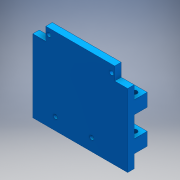
# Autodesk Inventor part: arduinoPlate
Saved by Autodesk Inventor 2016 (Build 200138000, 138)
## iProperties
Created: 2016-06-12
Part Number: arduinoPlate
Material: ABS Plastic
Document SubType Name: Modeling
Designer: hesaon
Density: 1.06 g/cm^3
Appearance: Smooth - White
Author: hesaon
Autodesk Inventor part; units mm, degrees
ref_plane "YZ Plane" through (0, 0, 0) normal (1, 0, 0) x (0, 1, 0)
ref_plane "XZ Plane" through (0, 0, 0) normal (0, 1, 0) x (-1, 0, 0)
ref_plane "XY Plane" through (0, 0, 0) normal (0, 0, 1) x (1, 0, 0)
sketch "Sketch1" plane through (0, 0, 0) normal (0, 1, 0) x (-1, 0, 0)
  line L0 (0, 0) -> (73, 0)
  line L1 (73, 0) -> (73, -56)
  line L2 (73, -56) -> (0, -56)
  line L3 (0, -56) -> (0, 0)
  dimension "d0" = 73
  dimension "d1" = 56
  constraints: 8 end point, 2 parallel, 1 horizontal, 1 perpendicular
  measures "d0" distance of L1.end L2.end
  measures "d1" distance of L0.end L1.end
extrude "Extrusion1" add sketch "Sketch1" along normal blind 5
sketch "Sketch2" plane through (0, 5, 0) normal (0, 1, 0) x (1, 0, 0)
  line L0 (-73, 46) -> (-63, 46)
  line L1 (-63, 46) -> (-63, 36)
  line L2 (-63, 36) -> (-73, 36)
  line L3 (-73, 36) -> (-73, 46)
  line L4 (-10, 46) -> (0, 46)
  line L5 (0, 46) -> (0, 36)
  line L6 (0, 36) -> (-10, 36)
  line L7 (-10, 36) -> (-10, 46)
  line L8 (-73, 20) -> (-63, 20)
  line L9 (-63, 20) -> (-63, 10)
  line L10 (-63, 10) -> (-73, 10)
  line L11 (-73, 10) -> (-73, 20)
  line L12 (-10, 20) -> (0, 20)
  line L13 (0, 20) -> (0, 10)
  line L14 (0, 10) -> (-10, 10)
  line L15 (-10, 10) -> (-10, 20)
  line L16 (-73, 56) -> (-73, 0) projected
  line L17 (0, 0) -> (0, 56) projected
  line L18 (0, 56) -> (-73, 56) projected
  line L19 (-73, 0) -> (0, 0) projected
  dimension "d4" = 10
  dimension "d5" = 10
  dimension "d6" = 10
  dimension "d7" = 10
  dimension "d8" = 10
  dimension "d9" = 10
  dimension "d10" = 10
  dimension "d11" = 10
  dimension "d12" = 10
  dimension "d13" = 10
  dimension "d14" = 10
  dimension "d15" = 10
  constraints: 32 end point, 8 parallel, 4 collinear, 4 horizontal, 4 perpendicular
  measures "d4" distance of L1.end L2.end
  measures "d5" distance of L0.end L1.end
  measures "d6" distance of L5.end L6.end
  measures "d7" distance of L4.end L5.end
  measures "d8" distance of L9.end L10.end
  measures "d9" distance of L8.end L9.end
  measures "d10" distance of L13.end L14.end
  measures "d11" distance of L12.end L13.end
  measures "d12" distance between parallel lines of L18 L0
  measures "d13" distance between parallel lines of L19 L10
  measures "d14" distance between parallel lines of L19 L14
  measures "d15" distance between parallel lines of L18 L4
extrude "Extrusion2" add sketch "Sketch2" along normal blind 10 contours L0 L1 L2 L3 | L8 L9 L10 L11 | L5 L6 L7 L4 | L13 L14 L15 L12
hole "Hole1" at (-68, 10, -46) direction (0, 0, 1) diameter 4.3 end through all
hole "Hole2" at (-5, 10, -46) direction (0, 0, 1) diameter 4.3 end through all
sketch "Sketch4" plane through (0, 0, 0) normal (0, -1, 0) x (1, 0, 0)
  line L0 (-63.15, 19.6) -> (-9.85, 19.6)
  line L1 (-9.85, 19.6) -> (-9.85, -49)
  line L2 (-9.85, -49) -> (-63.15, -49)
  line L3 (-63.15, -49) -> (-63.15, 19.6)
  line L4 (0, -56) -> (-73, -56) projected
  line L5 (-73, 0) -> (-73, -56) projected
  circle A0 centre (-55.55, -46.5) radius 1.6
  circle A1 centre (-27.65, -46.5) radius 1.6
  circle A2 centre (-12.45, 4.3) radius 1.6
  circle A3 centre (-60.65, 5.6) radius 1.6
  point P0 (0, 0)
  dimension "d40" = 53.3
  dimension "d41" = 68.6
  dimension "d42" = 7
  dimension "d43" = 9.85
  dimension "d44" = 3.2
  dimension "d45" = 3.2
  dimension "d46" = 3.2
  dimension "d47" = 3.2
  dimension "d48" = 14
  dimension "d49" = 15.3
  dimension "d50" = 2.5
  dimension "d51" = 7.6
  dimension "d52" = 66.1
  dimension "d53" = 66.1
  dimension "d54" = 27.9
  dimension "d55" = 15.2
  constraints: 8 end point, 4 centre point, 2 parallel, 1 horizontal, 1 perpendicular
  measures "d40" distance of L1.end L2.end
  measures "d41" distance of L0.end L1.end
  measures "d42" distance between parallel lines of L4 L2
  measures "d43" distance between parallel lines of L5 L3
  measures "d44" diameter of A0
  measures "d45" diameter of A1
  measures "d46" diameter of A2
  measures "d47" diameter of A3
  measures "d48" distance from line of L0 A3.centre
  measures "d49" distance from line of L0 A2.centre
  measures "d50" distance from line of L3 A3.centre
  measures "d51" distance from line of L3 A0.centre
  measures "d52" distance from line of L0 A0.centre
  measures "d53" distance from line of L0 A1.centre
  measures "d54" distance of A0.centre A1.centre
  measures "d55" horizontal distance of A1.centre A2.centre
sketch "Sketch5" plane through (-73, 0, 0) normal (0, 0, 1) x (1, 0, 0)
  line L0 (10, 5) -> (63, 5)
  line L1 (63, 5) -> (63, 0)
  line L2 (63, 0) -> (10, 0)
  line L3 (10, 0) -> (10, 5)
  line L4 (73, 0) -> (0, 0) projected
  line L5 (0, 5) -> (73, 5) projected
  line L6 (73, 0) -> (73, 5) projected
  dimension "d56" = 10
  dimension "d57" = 10
  constraints: 8 end point, 2 collinear, 2 parallel, 1 horizontal, 1 perpendicular
  measures "d56" distance of L5.start L0.start
  measures "d57" distance between parallel lines of L6 L1
extrude "Extrusion3" add sketch "Sketch5" along normal blind 10 contours L0 L1 L2 L3
extrude "Extrusion4" cut sketch "Sketch4" against normal up to next contours A0 | A1 | A2 | A3
body "Solid1"
